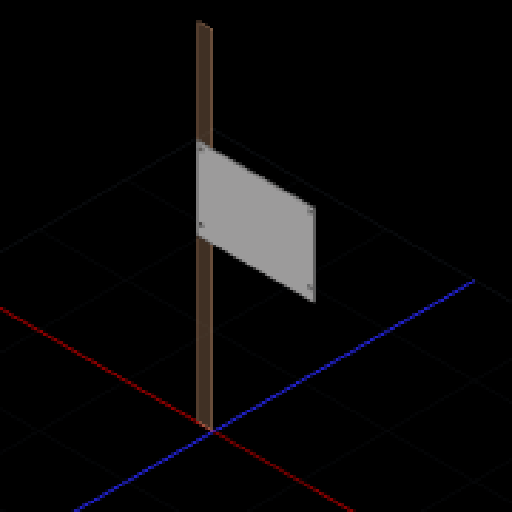
# Autodesk Inventor part: bottom rails
Saved by Autodesk Inventor 2025.2 (Build 292293000, 293)
## iProperties
Created: 2026-01-16
Part Number: bottom rails
Material: Acetal Resin, Black
Document SubType Name: Modeling
Designer: cloudy
Density: 1.425 g/cm^3
Appearance: Smooth - Black
Author: cloudy
Autodesk Inventor part; units mm, degrees
ref_plane "YZ Plane" through (0, 0, 0) normal (1, 0, 0) x (0, 1, 0)
ref_plane "XZ Plane" through (0, 0, 0) normal (0, 1, 0) x (-1, 0, 0)
ref_plane "XY Plane" through (0, 0, 0) normal (0, 0, 1) x (1, 0, 0)
ref_plane "Work Plane1" through (0, 0, 0) normal (0, 0, 1) x (1, 0, 0)
sketch "Sketch1" plane through (228.6, 0, 0) normal (0, 0, -1) x (-1, 0, 0)
  circle A0 centre (-12.7, 0) radius 2.1971 projected
  circle A1 centre (114.3, 0) radius 2.1971 projected
  circle A2 centre (-12.7, 76.2) radius 2.1971 projected
  circle A3 centre (114.3, 76.2) radius 2.1971 projected
  line L0 (-17.78, 120.65) -> (119.38, 120.65)
  line L1 (119.38, 120.65) -> (119.38, -12.7)
  line L2 (119.38, -12.7) -> (-17.78, -12.7)
  line L3 (-17.78, -12.7) -> (-17.78, 120.65)
  circle A4 centre (114.3, 114.3) radius 2.1844 projected
  circle A5 centre (-12.7, 114.3) radius 2.1844 projected
  point P0 (228.6, 0)
  dimension "d0" = 12.7
  dimension "d2" = 5.08
  dimension "d3" = 5.08
  dimension "d6" = 6.35
  constraints: 8 end point, 2 parallel, 1 horizontal, 1 perpendicular
  measures "d0" distance from line of L2 A1.centre
  measures "d2" distance from line of L1 A3.centre
  measures "d3" distance from line of L3 A2.centre
  measures "d6" distance from line of L0 A4.centre
extrude "Extrusion1" add sketch "Sketch1" along normal blind 1.5
fillet "Fillet2" radius 5.715 4 edges at (246.38, 120.65, -0.75) (109.22, 120.65, -0.75) (109.22, -12.7, -0.75) (246.38, -12.7, -0.75)
sketch "Sketch7" plane through (109.22, -6.985, 0) normal (-1, 0, 0) x (0, 0, 1)
  circle A0 centre (-9.3619, 102.3193) radius 2.2479 projected
  arc A1 (-12.6628, 105.7523) -> (-12.0724, 98.4034) centre (-9.3619, 102.3193) ccw
  line L0 (-12.6628, 105.7523) -> (-1.5, 116.4856)
  line L1 (-12.0724, 98.4034) -> (-1.5, 91.0856)
  line L2 (-1.5, 0) -> (-1.5, 121.92) projected
  point P0 (0, 6.985)
  dimension "d38" = 9.525
  dimension "d39" = 25.4
  dimension "d40" = 78.566
  constraints: 4 end point, 2 point on circle, 2 point on line, 2 tangent, 1 centre point, 1 coincident
  measures "d38" diameter of A1
  measures "d39" distance of L0.end L1.end
  measures "d40" angle of L0 L1
extrude "Extrusion6" add sketch "Sketch7" against normal up to surface (137.16 mm away)
sketch "Sketch8" plane through (228.6, 0, -1.5) normal (0, 0, -1) x (-1, 0, 0)
  arc A0 (-17.78, -6.985) -> (-12.065, -12.7) centre (-12.065, -6.985) ccw projected
  line L0 (-17.78, 114.935) -> (-17.78, -6.985) projected
  arc A1 (-12.065, 120.65) -> (-17.78, 114.935) centre (-12.065, 114.935) ccw projected
  line L1 (113.665, 120.65) -> (-12.065, 120.65) projected
  arc A2 (119.38, 114.935) -> (113.665, 120.65) centre (113.665, 114.935) ccw projected
  line L2 (119.38, -6.985) -> (119.38, 114.935) projected
  arc A3 (113.665, -12.7) -> (119.38, -6.985) centre (113.665, -6.985) ccw projected
  line L3 (-12.065, -12.7) -> (113.665, -12.7) projected
  circle A4 centre (-12.7, 114.3) radius 2.1844 projected
  circle A5 centre (114.3, 114.3) radius 2.1844 projected
  circle A6 centre (114.3, 76.2) radius 2.1971 projected
  circle A7 centre (-12.7, 76.2) radius 2.1971 projected
  circle A8 centre (114.3, 0) radius 2.1971 projected
  circle A9 centre (-12.7, 0) radius 2.1971 projected
  line L4 (119.38, 84.1006) -> (-17.78, 84.1006) projected
  line L5 (-17.78, 109.5006) -> (119.38, 109.5006) projected
  line L6 (-12.7, 109.5006) -> (-12.7, 84.1006)
  line L7 (114.3, 84.1006) -> (114.3, 109.5006)
  point P0 (228.6, 0)
  dimension "d43" = 5.08
  dimension "d44" = 5.08
  constraints: 4 end point, 4 point on line, 2 vertical
  measures "d43" distance between parallel lines of L2 L7
  measures "d44" distance between parallel lines of L0 L6
extrude "Extrusion7" cut sketch "Sketch8" along normal through all contours L6 L5 L7 L4
chamfer "Chamfer2" distance 3.175 angle 45 2 edges at (114.3, 96.8006, -1.5) (241.3, 96.8006, -1.5)
sketch "Sketch9" plane through (228.6, 0, -1.5) normal (0, 0, -1) x (-1, 0, 0)
  line L0 (113.665, 120.65) -> (-12.065, 120.65) projected
  line L1 (-6.35, 120.65) -> (107.95, 120.65)
  line L2 (107.95, 120.65) -> (107.95, 82.55)
  line L3 (107.95, 82.55) -> (-6.35, 82.55)
  line L4 (-6.35, 82.55) -> (-6.35, 120.65)
  line L5 (119.38, -6.985) -> (119.38, 84.1006) projected
  line L6 (-17.78, 84.1006) -> (-17.78, -6.985) projected
  point P0 (228.6, 0)
  dimension "d50" = 38.1
  dimension "d51" = 114.3
  dimension "d52" = 11.43
  dimension "d53" = 11.43
  constraints: 8 end point, 2 parallel, 1 horizontal, 1 perpendicular, 1 point on line
  measures "d50" distance of L1.end L2.end
  measures "d51" distance of L2.end L3.end
  measures "d52" distance between parallel lines of L5 L2
  measures "d53" distance between parallel lines of L6 L4
extrude "Extrusion8" cut sketch "Sketch9" against normal through all
fillet "Fillet3" radius 5.715 4 edges at (234.95, 82.55, -0.75) (120.65, 82.55, -0.75) (120.65, 120.65, -0.75) (234.95, 120.65, -0.75)
equation "\"d52\" = d53"
body "Solid1"
